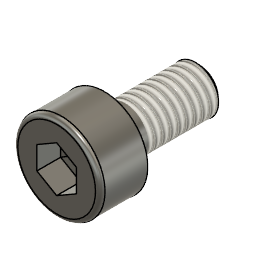
Tachometer (Autodesk Fusion 360 archive; units mm, degrees)
design "Forged Hexagon Socket Head Cap Screw ANSI B18.3.1M - M3x0.5 x 6 Steel Grade 2 Plain"
description: Forged Hexagon Socket Head Cap Screw ANSI B18.3.1M - M3x0.5 x 6
part number: FSHCS ANSI B18.3.1M - M3x0.5 x 6 Steel Grade 2 Plain
Autodesk Fusion 360 part; units mm, degrees
sketch "Sketch1" plane through (0, 0, 0) normal (0, 1, 0) x (1, 0, 0)
  line L0 (-1.5, 0) -> (-1.5, 6)
  line L1 (-1.5, 6) -> (0, 6)
  line L2 (0, 6) -> (0, -3)
  line L3 (-1.5, 0) -> (-2.75, 0)
  line L4 (-2.75, 0) -> (-2.75, -3)
  line L5 (-2.75, -3) -> (0, -3)
  dimension "d101" = 6
  dimension "d102" = 3
  dimension "d109" = 5.5
  dimension "d110" = 3
  constraint perpendicular L0 L1
  constraint collinear origin L1.end L2.end
  constraint perpendicular L0 L3
  constraint coincident origin L3
  constraint vertical L2
  constraint coincident L2 L5.end
  constraint perpendicular L2 L5
  measures "d101" distance of origin L1
  measures "d102" distance of L3.end L5
revolve "Revolve1" add sketch "Sketch1" angle 360 about axis through (0, 0, -6) along (0, 0, 1)
ref_plane "WorkPlane1" through (0, 0, 3) normal (0, 0, 1) x (1, 0, 0)
sketch "Sketch6" plane through (0, 0, 3) normal (0, 0, 1) x (1, 0, 0)
  line L0 (0, -1.4434) -> (1.25, -0.7217)
  line L1 (1.25, -0.7217) -> (1.25, 0.7217)
  line L2 (1.25, 0.7217) -> (0, 1.4434)
  line L3 (0, 1.4434) -> (-1.25, 0.7217)
  line L4 (-1.25, 0.7217) -> (-1.25, -0.7217)
  line L5 (-1.25, -0.7217) -> (0, -1.4434)
  dimension "d111" = 2.5
  constraint vertical L1
  measures "d111" distance of L1 L4
extrude "Extrude1" cut sketch "Sketch6" against normal blind 1.5
extrude "Extrude2" cut 1 faces at (0.4167, -0.2406, 1.5) along direction (0, 0, -1) blind 1.5 draft -85
thread "Thread3" "ANSI Metric M Profile 3.0 M3x0.5 M3x0.5 4g6g" major diameter 2.927 minor diameter 2.369 pitch 0.5 angle 60 resizes the face on face at (-1.4925, 0.1494, -4) from (0, 0, -1.3067) to (0, 0, -6)
fillet "Fillet4" radius 0.3 1 edges at (-2.5639, 0.9944, 3)
sketch "Sketch7" plane through (0, 0, 0) normal (0, 1, 0) x (1, 0, 0)
  line L0 (-1.53, 6) -> (-1.53, 5.6933)
  line L1 (-1.53, 5.6933) -> (-1.1933, 6)
  line L2 (0, 6) -> (0, -3)
  line L3 (-1.53, 6) -> (0, 6)
  dimension "d104" = 1.1933
  dimension "d105" = 1.53
  dimension "d106" = 0.3067
  constraint coincident L2.start L3.end
  constraint perpendicular L2 L3
  constraint coincident L1.end L3
  constraint perpendicular L0 L3
  measures "d104" distance of L1.end L2
  measures "d105" distance of L0 L2.start
  measures "d106" distance of L0.end L3
revolve "Revolve3" cut sketch "Sketch7" angle 360 about axis through (0, 0, 1.75) along (0, 0, 1)
equation "adsk_nomlen = 6.00 mm"
equation "adsk_headh = 3.00 mm"
equation "adsk_headdia = 5.50 mm"
equation "adsk_nomdia = 3.00 mm"
equation "adsk_philwidth = 2.50 mm"
equation "d31 = -adsk_phildepth"
equation "adsk_phildepth = 1.50 mm"
equation "d71 = adsk_headh"
equation "d76 = -adsk_phildepth"
equation "adsk_thrlen = 4.693275 mm"
equation "d86 = adsk_nomdia * 0.1"
equation "adsk_startlen = 0.306725 mm"
equation "adsk_endpointdia = 2.38655 mm"
equation "d101 = adsk_nomlen"
equation "d102 = adsk_headh"
equation "d104 = adsk_endpointdia / 2"
equation "d105 = adsk_nomdia * 0.51"
equation "d106 = adsk_startlen"
equation "d108 = min(adsk_thrlen; adsk_nomlen - 0.001 mm)"
equation "d109 = adsk_headdia"
equation "d110 = adsk_nomdia"
equation "d111 = adsk_philwidth"

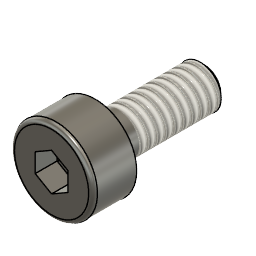
design "Broached Hexagon Socket Head Cap Screw ANSI B18.3.1M - M2x0.4 x 5 Steel Grade 2 Plain"
description: Broached Hexagon Socket Head Cap Screw ANSI B18.3.1M - M2x0.4 x 5
part number: BSHCS ANSI B18.3.1M - M2x0.4 x 5 Steel Grade 2 Plain
Autodesk Fusion 360 part; units mm, degrees
sketch "Sketch1" plane through (0, 0, 0) normal (0, 1, 0) x (1, 0, 0)
  line L0 (-1, 0) -> (-1, 5)
  line L1 (-1, 5) -> (0, 5)
  line L2 (0, 5) -> (0, -2)
  line L3 (-1, 0) -> (-1.9, 0)
  line L4 (-1.9, 0) -> (-1.9, -2)
  line L5 (-1.9, -2) -> (0, -2)
  dimension "d101" = 5
  dimension "d102" = 2
  dimension "d109" = 3.8
  dimension "d110" = 2
  constraint perpendicular L0 L1
  constraint collinear origin L1.end L2.end
  constraint perpendicular L0 L3
  constraint coincident origin L3
  constraint vertical L2
  constraint coincident L2 L5.end
  constraint perpendicular L2 L5
  measures "d101" distance of origin L1
  measures "d102" distance of L3.end L5
revolve "Revolve1" add sketch "Sketch1" angle 360 about axis through (0, 0, -5) along (0, 0, 1)
ref_plane "WorkPlane1" through (0, 0, 2) normal (0, 0, 1) x (1, 0, 0)
sketch "Sketch6" plane through (0, 0, 2) normal (0, 0, 1) x (1, 0, 0)
  line L0 (0, -0.866) -> (0.75, -0.433)
  line L1 (0.75, -0.433) -> (0.75, 0.433)
  line L2 (0.75, 0.433) -> (0, 0.866)
  line L3 (0, 0.866) -> (-0.75, 0.433)
  line L4 (-0.75, 0.433) -> (-0.75, -0.433)
  line L5 (-0.75, -0.433) -> (0, -0.866)
  dimension "d111" = 1.5
  constraint vertical L1
  measures "d111" distance of L1 L4
extrude "Extrude1" cut sketch "Sketch6" against normal blind 1
extrude "Extrude2" cut 1 faces at (0, -0.2887, 1) along direction (0, 0, -1) blind 1 draft -85
thread "Thread3" "ANSI Metric M Profile 2.0 M2x0.4 M2x0.4 4g6g" major diameter 1.9335 minor diameter 1.4905 pitch 0.4 angle 60 resizes the face on face at (-0.9988, 0.0498, -3.3333) from (0, 0, -1.0454) to (0, 0, -5)
fillet "Fillet4" radius 0.2 1 edges at (-1.7714, 0.6871, 2)
sketch "Sketch7" plane through (0, 0, 0) normal (0, 1, 0) x (1, 0, 0)
  line L0 (-1.02, 5) -> (-1.02, 4.7546)
  line L1 (-1.02, 4.7546) -> (-0.7546, 5)
  line L2 (0, 5) -> (0, -2)
  line L3 (-1.02, 5) -> (0, 5)
  dimension "d104" = 0.7546
  dimension "d105" = 1.02
  dimension "d106" = 0.2454
  constraint coincident L2.start L3.end
  constraint perpendicular L2 L3
  constraint coincident L1.end L3
  constraint perpendicular L0 L3
  measures "d104" distance of L1.end L2
  measures "d105" distance of L0 L2.start
  measures "d106" distance of L0.end L3
revolve "Revolve3" cut sketch "Sketch7" angle 360 about axis through (0, 0, 1.75) along (0, 0, 1)
equation "adsk_nomlen = 5.00 mm"
equation "adsk_headh = 2.00 mm"
equation "adsk_headdia = 3.80 mm"
equation "adsk_nomdia = 2.00 mm"
equation "adsk_philwidth = 1.50 mm"
equation "d31 = -adsk_phildepth"
equation "adsk_phildepth = 1.00 mm"
equation "d71 = adsk_headh"
equation "d76 = -adsk_phildepth"
equation "adsk_thrlen = 3.95462 mm"
equation "d86 = adsk_nomdia * 0.1"
equation "adsk_startlen = 0.24538 mm"
equation "adsk_endpointdia = 1.50924 mm"
equation "d101 = adsk_nomlen"
equation "d102 = adsk_headh"
equation "d104 = adsk_endpointdia / 2"
equation "d105 = adsk_nomdia * 0.51"
equation "d106 = adsk_startlen"
equation "d108 = min(adsk_thrlen; adsk_nomlen - 0.001 mm)"
equation "d109 = adsk_headdia"
equation "d110 = adsk_nomdia"
equation "d111 = adsk_philwidth"

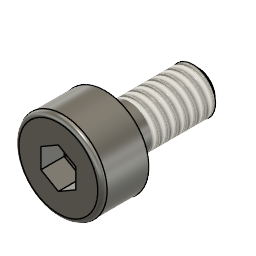
design "Broached Hexagon Socket Head Cap Screw ANSI B18.3.1M - M2x0.4 x 4 Steel Grade 2 Plain"
description: Broached Hexagon Socket Head Cap Screw ANSI B18.3.1M - M2x0.4 x 4
part number: BSHCS ANSI B18.3.1M - M2x0.4 x 4 Steel Grade 2 Plain
Autodesk Fusion 360 part; units mm, degrees
sketch "Sketch1" plane through (0, 0, 0) normal (0, 1, 0) x (1, 0, 0)
  line L0 (-1, 0) -> (-1, 4)
  line L1 (-1, 4) -> (0, 4)
  line L2 (0, 4) -> (0, -2)
  line L3 (-1, 0) -> (-1.9, 0)
  line L4 (-1.9, 0) -> (-1.9, -2)
  line L5 (-1.9, -2) -> (0, -2)
  dimension "d101" = 4
  dimension "d102" = 2
  dimension "d109" = 3.8
  dimension "d110" = 2
  constraint perpendicular L0 L1
  constraint collinear origin L1.end L2.end
  constraint perpendicular L0 L3
  constraint coincident origin L3
  constraint vertical L2
  constraint coincident L2 L5.end
  constraint perpendicular L2 L5
  measures "d101" distance of origin L1
  measures "d102" distance of L3.end L5
revolve "Revolve1" add sketch "Sketch1" angle 360 about axis through (0, 0, -4) along (0, 0, 1)
ref_plane "WorkPlane1" through (0, 0, 2) normal (0, 0, 1) x (1, 0, 0)
sketch "Sketch6" plane through (0, 0, 2) normal (0, 0, 1) x (1, 0, 0)
  line L0 (0, -0.866) -> (0.75, -0.433)
  line L1 (0.75, -0.433) -> (0.75, 0.433)
  line L2 (0.75, 0.433) -> (0, 0.866)
  line L3 (0, 0.866) -> (-0.75, 0.433)
  line L4 (-0.75, 0.433) -> (-0.75, -0.433)
  line L5 (-0.75, -0.433) -> (0, -0.866)
  dimension "d111" = 1.5
  constraint vertical L1
  measures "d111" distance of L1 L4
extrude "Extrude1" cut sketch "Sketch6" against normal blind 1
extrude "Extrude2" cut 1 faces at (0, -0.2887, 1) along direction (0, 0, -1) blind 1 draft -85
thread "Thread3" "ANSI Metric M Profile 2.0 M2x0.4 M2x0.4 4g6g" major diameter 1.9335 minor diameter 1.4905 pitch 0.4 angle 60 resizes the face on face at (-0.9988, 0.0498, -2.6667) from (0, 0, -1.0454) to (0, 0, -4)
fillet "Fillet4" radius 0.2 1 edges at (-1.7714, 0.6871, 2)
sketch "Sketch7" plane through (0, 0, 0) normal (0, 1, 0) x (1, 0, 0)
  line L0 (-1.02, 4) -> (-1.02, 3.7546)
  line L1 (-1.02, 3.7546) -> (-0.7546, 4)
  line L2 (0, 4) -> (0, -2)
  line L3 (-1.02, 4) -> (0, 4)
  dimension "d104" = 0.7546
  dimension "d105" = 1.02
  dimension "d106" = 0.2454
  constraint coincident L2.start L3.end
  constraint perpendicular L2 L3
  constraint coincident L1.end L3
  constraint perpendicular L0 L3
  measures "d104" distance of L1.end L2
  measures "d105" distance of L0 L2.start
  measures "d106" distance of L0.end L3
revolve "Revolve3" cut sketch "Sketch7" angle 360 about axis through (0, 0, 1.75) along (0, 0, 1)
equation "adsk_nomlen = 4.00 mm"
equation "adsk_headh = 2.00 mm"
equation "adsk_headdia = 3.80 mm"
equation "adsk_nomdia = 2.00 mm"
equation "adsk_philwidth = 1.50 mm"
equation "d31 = -adsk_phildepth"
equation "adsk_phildepth = 1.00 mm"
equation "d71 = adsk_headh"
equation "d76 = -adsk_phildepth"
equation "adsk_thrlen = 2.95462 mm"
equation "d86 = adsk_nomdia * 0.1"
equation "adsk_startlen = 0.24538 mm"
equation "adsk_endpointdia = 1.50924 mm"
equation "d101 = adsk_nomlen"
equation "d102 = adsk_headh"
equation "d104 = adsk_endpointdia / 2"
equation "d105 = adsk_nomdia * 0.51"
equation "d106 = adsk_startlen"
equation "d108 = min(adsk_thrlen; adsk_nomlen - 0.001 mm)"
equation "d109 = adsk_headdia"
equation "d110 = adsk_nomdia"
equation "d111 = adsk_philwidth"
